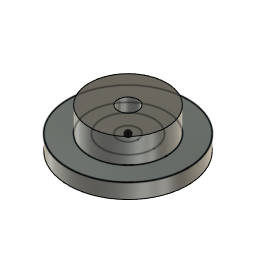
EggBot Axis Support (Autodesk Fusion 360 design; units mm, degrees)
Autodesk Fusion 360 part; units mm, degrees
sketch "Sketch1" plane through (0, 0, 0) normal (0, 0, 1) x (1, 0, 0)
  circle A0 centre (0, 0) radius 7.75
  circle A1 centre (0, 0) radius 12
  circle A2 centre (0, 0) radius 2
  circle A3 centre (0, 0) radius 5.2
  dimension "d1" = 15.5
  dimension "d2" = 24
  dimension "d3" = 4
  dimension "d4" = 10.4
  constraint coincident A0.centre A1.centre
  constraint concentric A0 A1
  constraint concentric A0 A2
  measures "d1" diameter of A0
  measures "d2" diameter of A1
  measures "d3" diameter of A2
  measures "d4" diameter of A3
extrude "Extrude1" add sketch "Sketch1" along normal blind 5 contours A0 | A3
extrude "Extrude2" add sketch "Sketch1" against normal blind 3 contours A0 | A1
